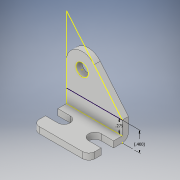
# Autodesk Inventor part: PinAtttachments
Saved by Autodesk Inventor 2018 (Build 220112000, 112)
## iProperties
Created: 2020-02-07
Part Number: PinAtttachments
Material: Generic
Document SubType Name: Modeling
Designer: JMHal
Density: 1 g/cm^3
Appearance: Default
Author: JMHal
Autodesk Inventor part; units mm, degrees
ref_plane "YZ Plane" through (0, 0, 0) normal (1, 0, 0) x (0, 1, 0)
ref_plane "XZ Plane" through (0, 0, 0) normal (0, 1, 0) x (-1, 0, 0)
ref_plane "XY Plane" through (0, 0, 0) normal (0, 0, 1) x (1, 0, 0)
sketch "Sketch1" plane through (0, 0, 0) normal (0, 1, 0) x (-1, 0, 0)
  line L0 (0, 0) -> (28.575, 0)
  line L1 (28.575, 0) -> (28.575, -20.32)
  line L2 (28.575, -20.32) -> (0, -20.32)
  line L3 (0, -20.32) -> (0, 0)
  dimension "d0" = 28.575
  dimension "d1" = 20.32
  constraints: 8 end point, 2 parallel, 1 horizontal, 1 perpendicular
  measures "d0" distance of L1.end L2.end
  measures "d1" distance of L0.end L1.end
extrude "Extrusion1" add sketch "Sketch1" along normal blind 3.175
fillet "Fillet1" radius 3.175 1 edges at (-14.2875, 0, -20.32)
fillet "Fillet2" radius 3.175 1 edges at (0, 1.5875, 0)
fillet "Fillet3" radius 3.175 1 edges at (-28.575, 1.5875, 0)
sketch "Sketch2" plane through (0, 3.175, 0) normal (0, 1, 0) x (1, 0, 0)
  line L0 (-28.575, 20.32) -> (-28.575, 3.175) projected
  line L1 (0, 3.175) -> (0, 20.32) projected
  line L2 (-28.575, 20.32) -> (0, 20.32)
  line L3 (0, 20.32) -> (0, 17.145)
  line L4 (0, 17.145) -> (-28.575, 17.145)
  line L5 (-28.575, 17.145) -> (-28.575, 20.32)
  point P0 (0, 0)
  dimension "d7" = 3.175
  constraints: 8 end point, 2 parallel, 1 horizontal, 1 perpendicular, 1 point on line
  measures "d7" distance between parallel lines of L2 L4
extrude "Extrusion2" add sketch "Sketch2" along normal blind 6.985
sketch "Sketch3" plane through (0, 3.175, 0) normal (0, 1, 0) x (1, 0, 0)
  line L0 (0, 17.145) -> (0, 3.175) projected
  line L1 (0, 6.35) -> (-6.35, 6.35)
  line L2 (-6.35, 6.35) -> (-6.35, 12.7)
  line L3 (-6.35, 12.7) -> (0, 12.7)
  line L4 (0, 12.7) -> (0, 6.35)
  line L5 (-28.575, 3.175) -> (-28.575, 17.145) projected
  line L6 (-28.575, 6.35) -> (-22.225, 6.35)
  line L7 (-22.225, 6.35) -> (-22.225, 12.7)
  line L8 (-22.225, 12.7) -> (-28.575, 12.7)
  line L9 (-28.575, 12.7) -> (-28.575, 6.35)
  line L10 (-25.4, 0) -> (-3.175, 0) projected
  line L11 (0, 20.32) -> (-28.575, 20.32) projected
  circle A0 centre (-6.35, 9.525) radius 3.175
  circle A1 centre (-22.225, 9.525) radius 3.175
  point P0 (0, 0)
  dimension "d10" = 6.35
  dimension "d11" = 7.62
  dimension "d12" = 6.35
  dimension "d13" = 6.35
  constraints: 16 end point, 4 parallel, 4 point on line, 2 horizontal, 2 midpoint, 2 perpendicular, 2 vertical alignment, 4 other
  measures "d10" distance between parallel lines of L10 L6
  measures "d11" distance between parallel lines of L11 L3
  measures "d12" distance between parallel lines of L5 L7
  measures "d13" distance between parallel lines of L0 L2
extrude "Extrusion3" cut sketch "Sketch3" against normal blind 25.4
sketch "Sketch4" plane through (-28.575, 3.175, -17.145) normal (0, 0, 1) x (1, 0, 0)
  line L0 (0, 0) -> (0, 6.985) projected
  line L1 (0, 6.985) -> (28.4507, 6.985)
  line L2 (28.575, 0) -> (0, 0) projected
  line L3 (28.575, -3.175) -> (0, -3.175) projected
  dimension "d16" = 6.985
  dimension "d17" = 10.16
  constraints: 2 end point
  measures "d16" distance from line of L2 L1.end
  measures "d17" distance from line of L3 L0.end
sketch "Sketch5" plane through (-28.575, 3.175, -17.145) normal (0, 0, 1) x (1, 0, 0)
  line L0 (28.575, 0) -> (28.575, 6.985) projected
  line L1 (28.575, 6.985) -> (0, 41.275)
  line L2 (28.575, -3.175) -> (0, -3.175) projected
  line L3 (0, 0) -> (0, 6.985) projected
  line L4 (28.575, 0) -> (0, 0) projected
  line L5 (0, 41.275) -> (0, 6.985)
  line L6 (0, 0) -> (0, 6.985) projected
  line L7 (0, 6.985) -> (28.575, 6.985)
  dimension "d18" = 44.45
  dimension "d19" = 0
  dimension "d20" = 6.985
  dimension "d21" = 6.985
  constraints: 6 end point, 2 point on line
  measures "d18" distance from line of L2 L1.end
  measures "d19" distance from line of L3 L1.end
  measures "d20" distance from line of L4 L1.start
  measures "d21" distance from line of L4 L5.end
extrude "Extrusion4" add sketch "Sketch5" against normal blind 3.175 contours L7 L5 L1
sketch "Sketch6" plane through (-28.575, 3.175, -17.145) normal (0, 0, 1) x (1, 0, 0)
  circle A0 centre (7.9375, 19.05) radius 3.175
  line L0 (28.575, -3.175) -> (0, -3.175) projected
  line L1 (0, 0) -> (0, 41.275) projected
  dimension "d24" = 22.225
  dimension "d25" = 7.9375
  dimension "d26" = 6.35
  constraints: 1 centre point
  measures "d24" distance from line of L0 A0.centre
  measures "d25" distance from line of L1 A0.centre
  measures "d26" diameter of A0
extrude "Extrusion5" cut sketch "Sketch6" against normal blind 3.175
sketch "Sketch7" plane through (-28.575, 3.175, -17.145) normal (0, 0, 1) x (1, 0, 0)
  line L0 (0, 0) -> (0, 41.275) projected
  line L1 (28.575, 6.985) -> (0, 41.275) projected
  circle A0 centre (7.9375, 19.05) radius 3.175 projected
  point P0 (28.575, -3.175)
fillet "Fillet4" radius 8.001 1 edges at (-28.575, 44.45, -18.7325)
body "Solid1"
